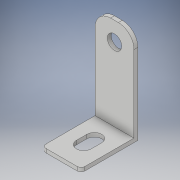
# Autodesk Inventor part: Angle bracket long
Saved by Autodesk Inventor 2018 (Build 220112000, 112)
## iProperties
Created: 2018-06-25
Part Number: Angle bracket long
Material: Generic
Document SubType Name: Modeling
Designer: Ajith Thomas
Density: 1 g/cm^3
Appearance: Default
Author: Ajith Thomas
Autodesk Inventor part; units mm, degrees
ref_plane "YZ Plane" through (0, 0, 0) normal (1, 0, 0) x (0, 1, 0)
ref_plane "XZ Plane" through (0, 0, 0) normal (0, 1, 0) x (-1, 0, 0)
ref_plane "XY Plane" through (0, 0, 0) normal (0, 0, 1) x (1, 0, 0)
sketch "Sketch1" plane through (0, 0, 0) normal (0, 1, 0) x (-1, 0, 0)
  line L0 (5, 7.3) -> (-5, 7.3)
  line L1 (-5, 7.3) -> (-5, -7.3)
  line L2 (-5, -7.3) -> (5, -7.3)
  line L3 (5, -7.3) -> (5, 7.3)
  line L4 (5, 7.3) -> (-5, -7.3) construction
  line L5 (-5, 7.3) -> (5, -7.3) construction
  point P0 (0, 0)
  dimension "d0" = 10
  dimension "d1" = 14.6
  constraints: 12 end point, 2 midpoint, 2 parallel, 1 horizontal, 1 perpendicular
  measures "d0" distance of L2.end L1.end
  measures "d1" distance of L1.end L0.end
extrude "Extrusion1" add sketch "Sketch1" along normal blind 1
sketch "Sketch2" plane through (5, 0, -7.3) normal (0, 0, -1) x (-1, 0, 0)
  line L0 (10, 0) -> (0, 0) projected
  line L1 (0, 0) -> (0, 24.7)
  line L2 (0, 24.7) -> (10, 24.7)
  line L3 (10, 24.7) -> (10, 0)
  point P0 (5, 0)
  dimension "d4" = 24.7
  constraints: 6 end point, 1 parallel, 1 perpendicular, 1 vertical
  measures "d4" distance of L0.end L1.end
extrude "Extrusion2" add sketch "Sketch2" against normal blind 1
fillet "Fillet1" radius 4 2 edges at (5, 24.7, -6.8) (-5, 24.7, -6.8)
fillet "Fillet2" radius 1 2 edges at (-5, 0.5, 7.3) (5, 0.5, 7.3)
sketch "Sketch3" plane through (5, 0, -7.3) normal (0, 0, -1) x (-1, 0, 0)
  circle A0 centre (5, 19.85) radius 1.85
  line L0 (0, 0) -> (0, 20.7) projected
  line L1 (5, 21.7) -> (6.6441, 21.7) construction
  line L2 (4, 24.7) -> (6, 24.7) construction
  point P0 (5, 0)
  dimension "d9" = 3.7
  dimension "d10" = 5
  dimension "d11" = 3
  constraints: 2 end point, 2 horizontal, 1 vertical alignment, 2 other
  measures "d10" distance from line of L0 point (5, 19.85)
  measures "d11" distance between parallel lines of L2 L1
extrude "Extrusion3" cut sketch "Sketch3" against normal blind 1
sketch "Sketch4" plane through (0, 0, 0) normal (0, -1, 0) x (1, 0, 0)
  arc A0 (1.9, 1.6) -> (-1.9, 1.6) centre (0, 1.6) ccw
  line L0 (-5, -7.3) -> (-5, 6.3) projected
  line L1 (-4, 7.3) -> (4, 7.3) construction
  line L2 (0, 3.5) -> (1.9, 3.5) construction
  arc A1 (-1.9, -1.1) -> (1.9, -1.1) centre (0, -1.1) ccw
  line L3 (0, -3) -> (1.9, -3) construction
  line L4 (1.9, 1.6) -> (1.9, -1.1)
  line L5 (-1.9, 1.6) -> (-1.9, -1.1)
  point P0 (0, 0)
  dimension "d14" = 3.8
  dimension "d15" = 5
  dimension "d17" = 3.8
  dimension "d18" = 3.8
  dimension "d19" = 6.5
  dimension "d20" = 5
  constraints: 8 end point, 6 point on circle, 5 tangent, 2 centre point, 2 horizontal
  measures "d14" diameter of A0
  measures "d15" distance from line of L0 A0.centre
  measures "d17" distance between parallel lines of L1 L2
  measures "d18" diameter of A1
  measures "d19" distance between parallel lines of L3 L2
  measures "d20" distance from line of L0 A1.centre
extrude "Extrusion4" cut sketch "Sketch4" against normal blind 1
body "Solid1"
